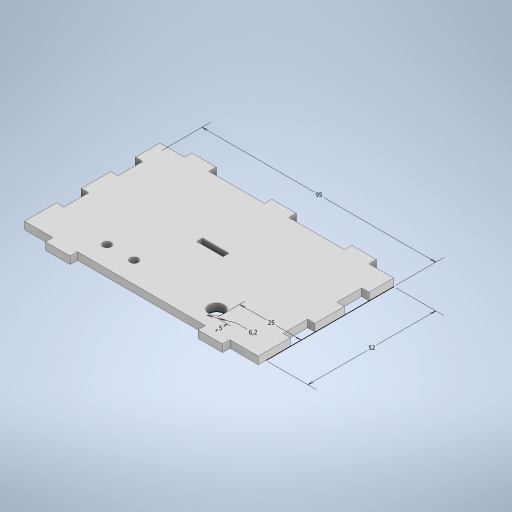
# Autodesk Inventor part: Parede_lateral_1
Saved by Autodesk Inventor 2024 (Build 280153000, 153)
## iProperties
Created: 2023-11-29
Part Number: Parede_lateral_1
Material: Genérico
Document SubType Name: Modeling
Designer: caiot
Density: 1 g/cm^3
Appearance: Padrão
Author: caiot
Autodesk Inventor part; units mm, degrees
ref_plane "YZ Plane" through (0, 0, 0) normal (1, 0, 0) x (0, 1, 0)
ref_plane "XZ Plane" through (0, 0, 0) normal (0, 1, 0) x (-1, 0, 0)
ref_plane "XY Plane" through (0, 0, 0) normal (0, 0, 1) x (1, 0, 0)
sketch "Parede_lateral_1" plane through (0, 0, 0) normal (0, 1, 0) x (-1, 0, 0)
  line L0 (0, 0) -> (-95, 0)
  line L1 (-95, 0) -> (-95, -52)
  line L2 (-95, -52) -> (0, -52)
  line L3 (0, -52) -> (0, 0)
  circle A0 centre (-70, -5) radius 3.1
  dimension "d0" = 95
  dimension "d1" = 52
  dimension "d101" = 6.2
  dimension "d102" = 5
  dimension "d105" = 25
  constraints: 8 end point, 2 parallel, 1 centre point, 1 horizontal, 1 perpendicular
  measures "d0" distance of L2.end L1.end
  measures "d1" distance of L1.end L0.end
  measures "d101" diameter of A0
  measures "d102" distance from line of L0 A0.centre
  measures "d105" distance from line of L1 A0.centre
extrude "Extrusão1" add sketch "Parede_lateral_1" along normal blind 3 contours L3 L2 L1 L0 | A0
sketch "Esboço3" plane through (0, 3, 0) normal (0, 1, 0) x (1, 0, 0)
  line L0 (42.1875, 27.15) -> (52.8125, 27.15)
  line L1 (52.8125, 27.15) -> (52.8125, 24.85)
  line L2 (52.8125, 24.85) -> (42.1875, 24.85)
  line L3 (42.1875, 24.85) -> (42.1875, 27.15)
  line L4 (95, 52) -> (0, 52) projected
  line L5 (95, 0) -> (95, 52) projected
  point P0 (0, 0)
  point P1 (46, 52)
  point P2 (27, 52)
  point P3 (47.5, 27.15)
  point P4 (95, 26)
  point P5 (52.8125, 26)
  dimension "d26" = 10.625
  dimension "d27" = 2.3
  dimension "d30" = 24.85
  dimension "d31" = 42.1875
  constraints: 8 end point, 3 midpoint, 2 parallel, 1 horizontal, 1 perpendicular
  measures "d26" distance of L1.end L2.end
  measures "d27" distance of L0.end L1.end
  measures "d30" distance from line of L4 point (47.5, 27.15)
  measures "d31" distance of point (95, 26) point (52.812, 26)
extrude "Extrusão3" cut sketch "Esboço3" against normal blind 10
sketch "Esboço4" plane through (0, 3, 0) normal (0, 1, 0) x (1, 0, 0)
  line L0 (95, 52) -> (0, 52) projected
  line L1 (0, 52) -> (0, 0) projected
  line L2 (10, 52) -> (20, 52)
  line L3 (20, 52) -> (20, 55)
  line L4 (20, 55) -> (10, 55)
  line L5 (10, 55) -> (10, 52)
  line L6 (42.5, 52) -> (52.5, 52)
  line L7 (52.5, 52) -> (52.5, 55)
  line L8 (52.5, 55) -> (42.5, 55)
  line L9 (42.5, 55) -> (42.5, 52)
  line L10 (75, 52) -> (85, 52)
  line L11 (85, 52) -> (85, 55)
  line L12 (85, 55) -> (75, 55)
  line L13 (75, 55) -> (75, 52)
  line L14 (0, 0) -> (95, 0) projected
  line L15 (95, 0) -> (95, 52) projected
  dimension "d43" = 3
  dimension "d74" = 3
  dimension "d75" = 3
  constraints: 24 end point, 6 parallel, 4 point on line, 3 horizontal, 3 perpendicular
  measures "d43" distance of L3.end L2.end
  measures "d74" distance between parallel lines of L8 L6
  measures "d75" distance between parallel lines of L12 L0
extrude "Extrusão4" add sketch "Esboço4" against normal blind 3 contours L0 L13 L12 L11 | L0 L9 L8 L7 | L5 L4 L3 L0
sketch "Esboço5" plane through (0, 3, 0) normal (0, 1, 0) x (1, 0, 0)
  line L0 (0, 10) -> (3, 10)
  line L1 (3, 10) -> (3, 20)
  line L2 (3, 20) -> (0, 20)
  line L3 (0, 20) -> (0, 10)
  line L4 (0, 32) -> (3, 32)
  line L5 (3, 32) -> (3, 42)
  line L6 (3, 42) -> (0, 42)
  line L7 (0, 42) -> (0, 32)
  line L8 (10, 52) -> (0, 52) projected
  line L9 (0, 0) -> (95, 0) projected
  line L10 (95, 0) -> (95, 52) projected
  line L11 (95, 10) -> (92, 10)
  line L12 (92, 10) -> (92, 20)
  line L13 (92, 20) -> (95, 20)
  line L14 (95, 20) -> (95, 10)
  line L15 (95, 42) -> (92, 42)
  line L16 (92, 42) -> (92, 32)
  line L17 (92, 32) -> (95, 32)
  line L18 (95, 32) -> (95, 42)
  line L19 (95, 52) -> (85, 52) projected
  line L20 (0, 0) -> (95, 0) projected
  point P0 (1.5, 42)
  point P1 (10, 0)
  point P2 (93.5, 42)
  point P3 (85, 0)
  point P4 (93.5, 10)
  point P5 (92, 37)
  point P6 (95, 37)
  dimension "d63" = 3
  dimension "d64" = 10
  dimension "d65" = 3
  dimension "d66" = 10
  dimension "d67" = 10
  dimension "d68" = 10
  dimension "d71" = 10
  dimension "d72" = 10
  dimension "d76" = 3
  dimension "d77" = 3
  constraints: 32 end point, 8 parallel, 5 midpoint, 4 horizontal, 4 perpendicular, 3 point on line
  measures "d63" distance of L2.end L1.end
  measures "d64" distance of L1.end L0.end
  measures "d65" distance of L6.end L5.end
  measures "d66" distance of L5.end L4.end
  measures "d67" distance from line of L8 point (1.5, 42)
  measures "d68" distance between parallel lines of L9 L0
  measures "d71" distance from line of L19 point (93.5, 42)
  measures "d72" distance from line of L20 point (93.5, 10)
  measures "d76" distance between parallel lines of L12 L10
  measures "d77" distance of point (92, 37) point (95, 37)
extrude "Extrusão5" cut sketch "Esboço5" against normal blind 3
sketch "Esboço6" plane through (0, 0, 0) normal (0, -1, 0) x (1, 0, 0)
  line L0 (0, 0) -> (95, 0)
  line L1 (95, 0) -> (95, 3)
  line L2 (95, 3) -> (0, 3)
  line L3 (0, 3) -> (0, 0)
  dimension "d79" = 95
  dimension "d80" = 3
  constraints: 8 end point, 2 parallel, 1 horizontal, 1 perpendicular
  measures "d79" distance of L2.end L1.end
  measures "d80" distance of L1.end L0.end
extrude "Extrusão6" add sketch "Esboço6" against normal blind 3
sketch "Esboço7" plane through (0, 0, 0) normal (0, -1, 0) x (1, 0, 0)
  line L0 (95, 3) -> (0, 3) projected
  line L1 (11.5, 3) -> (21.5, 3)
  line L2 (21.5, 3) -> (21.5, 6)
  line L3 (21.5, 6) -> (11.5, 6)
  line L4 (11.5, 6) -> (11.5, 3)
  line L5 (83.5, 3) -> (73.5, 3)
  line L6 (73.5, 3) -> (73.5, 6)
  line L7 (73.5, 6) -> (83.5, 6)
  line L8 (83.5, 6) -> (83.5, 3)
  line L9 (0, -10) -> (0, 3) projected
  line L10 (95, 3) -> (95, -10) projected
  point P0 (0, 0)
  point P1 (11.5, 4.5)
  point P2 (95, -3.5)
  point P3 (83.5, 4.5)
  point P4 (21.5, 3)
  dimension "d83" = 10
  dimension "d84" = 3
  dimension "d85" = 10
  dimension "d86" = 3
  dimension "d87" = 11.5
  dimension "d88" = 11.5
  constraints: 16 end point, 4 parallel, 3 midpoint, 2 horizontal, 2 perpendicular, 2 point on line
  measures "d83" distance of L3.end L2.end
  measures "d84" distance of L2.end L1.end
  measures "d85" distance of L6.end L7.end
  measures "d86" distance of L5.end L6.end
  measures "d87" distance from line of L9 point (11.5, 4.5)
  measures "d88" horizontal distance of point (95, -3.5) point (83.5, 4.5)
extrude "Extrusão7" add sketch "Esboço7" against normal blind 3
sketch "Esboço8" plane through (0, 3, 0) normal (0, 1, 0) x (1, 0, 0)
  circle A0 centre (25, 5.5) radius 1.6
  circle A1 centre (36, 5.5) radius 1.6
  line L0 (21.5, -3) -> (73.5, -3) projected
  line L1 (0, 10) -> (0, -3) projected
  point P0 (0, 0)
  dimension "d92" = 3.2
  dimension "d93" = 3.2
  dimension "d94" = 11
  dimension "d95" = 8.5
  dimension "d96" = 8.5
  dimension "d98" = 25
  constraints: 2 centre point
  measures "d92" diameter of A0
  measures "d93" diameter of A1
  measures "d94" distance of A0.centre A1.centre
  measures "d95" distance from line of L0 A0.centre
  measures "d96" distance from line of L0 A1.centre
  measures "d98" horizontal distance of point (0, 0) A0.centre
extrude "Extrusão8" cut sketch "Esboço8" against normal blind 10
extrude "Extrusão9" cut sketch "Parede_lateral_1" along normal blind 10 contours A0
equation "\"d30\" = -0.5 * d27 + 0.5 * d1"
equation "\"d31\" = -0.5 * d26 + 0.5 * d0"
